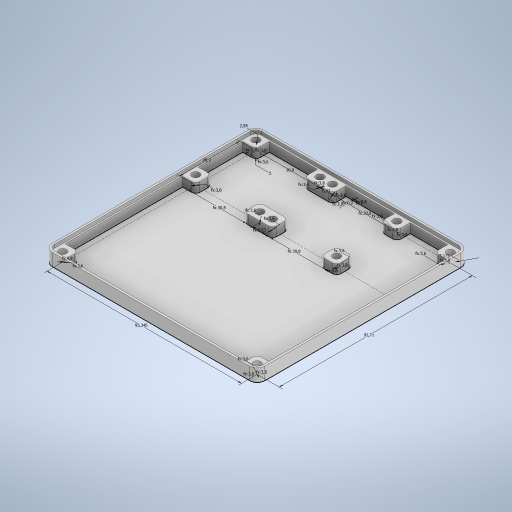
# Autodesk Inventor part: Housing_Bottom
Saved by Autodesk Inventor 2023 (Build 270158000, 158)
## iProperties
Created: 2023-02-18
Part Number: Housing_Bottom
Material: Generisch
Document SubType Name: Modeling
Designer: dvd62
Density: 1 g/cm^3
Appearance: Vorgabe
Author: dvd62
Autodesk Inventor part; units mm, degrees
ref_plane "YZ Plane" through (0, 0, 0) normal (1, 0, 0) x (0, 1, 0)
ref_plane "XZ Plane" through (0, 0, 0) normal (0, 1, 0) x (-1, 0, 0)
ref_plane "XY Plane" through (0, 0, 0) normal (0, 0, 1) x (1, 0, 0)
sketch "Skizze1" plane through (0, 0, 0) normal (0, 1, 0) x (-1, 0, 0)
  circle A0 centre (0, 0) radius 1.8
  line L0 (0, 0) -> (-93.345, 0) construction
  line L1 (-93.345, 0) -> (-93.345, -92.71) construction
  line L2 (-93.345, -92.71) -> (0, -92.71) construction
  line L3 (0, -92.71) -> (0, 0) construction
  circle A1 centre (0, -92.71) radius 1.8
  circle A2 centre (-93.345, -92.71) radius 1.8
  circle A3 centre (-93.345, 0) radius 1.8
  circle A4 centre (-30.8, -92.71) radius 1.8
  circle A5 centre (-36.83, -92.71) radius 1.8
  circle A6 centre (-67.63, -92.71) radius 1.8
  line L4 (0, -63.81) -> (-93.345, -63.81) construction
  circle A7 centre (0, -63.81) radius 1.8
  circle A8 centre (-30.8, -63.81) radius 1.8
  circle A9 centre (-36.83, -63.81) radius 1.8
  circle A10 centre (-67.63, -63.81) radius 1.8
  line L5 (0.635, -95.885) -> (-93.98, -95.885) construction
  line L6 (-96.52, -93.345) -> (-96.52, 0.635) construction
  line L7 (-93.98, 3.175) -> (0.635, 3.175) construction
  line L8 (3.175, 0.635) -> (3.175, -93.345) construction
  arc A11 (0.635, -95.885) -> (3.175, -93.345) centre (0.635, -93.345) ccw construction
  arc A12 (-96.52, -93.345) -> (-93.98, -95.885) centre (-93.98, -93.345) ccw construction
  arc A13 (-93.98, 3.175) -> (-96.52, 0.635) centre (-93.98, 0.635) ccw construction
  arc A14 (3.175, 0.635) -> (0.635, 3.175) centre (0.635, 0.635) ccw construction
  line L9 (-93.98, -96.085) -> (0.635, -96.085)
  arc A15 (0.635, -96.085) -> (3.375, -93.345) centre (0.635, -93.345) ccw
  line L10 (3.375, -93.345) -> (3.375, 0.635)
  arc A16 (3.375, 0.635) -> (0.635, 3.375) centre (0.635, 0.635) ccw
  line L11 (0.635, 3.375) -> (-93.98, 3.375)
  arc A17 (-93.98, 3.375) -> (-96.72, 0.635) centre (-93.98, 0.635) ccw
  line L12 (-96.72, 0.635) -> (-96.72, -93.345)
  arc A18 (-96.72, -93.345) -> (-93.98, -96.085) centre (-93.98, -93.345) ccw
  line L13 (0.635, -97.085) -> (-93.98, -97.085)
  arc A19 (-97.72, -93.345) -> (-93.98, -97.085) centre (-93.98, -93.345) ccw
  line L14 (-97.72, -93.345) -> (-97.72, 0.635)
  arc A20 (-93.98, 4.375) -> (-97.72, 0.635) centre (-93.98, 0.635) ccw
  line L15 (-93.98, 4.375) -> (0.635, 4.375)
  arc A21 (4.375, 0.635) -> (0.635, 4.375) centre (0.635, 0.635) ccw
  line L16 (4.375, 0.635) -> (4.375, -93.345)
  arc A22 (0.635, -97.085) -> (4.375, -93.345) centre (0.635, -93.345) ccw
  line L17 (0.635, -95.285) -> (-93.98, -95.285)
  arc A23 (-95.92, -93.345) -> (-93.98, -95.285) centre (-93.98, -93.345) ccw
  line L18 (-95.92, -93.345) -> (-95.92, 0.635)
  arc A24 (-93.98, 2.575) -> (-95.92, 0.635) centre (-93.98, 0.635) ccw
  line L19 (-93.98, 2.575) -> (0.635, 2.575)
  arc A25 (2.575, 0.635) -> (0.635, 2.575) centre (0.635, 0.635) ccw
  line L20 (2.575, 0.635) -> (2.575, -93.345)
  arc A26 (0.635, -95.285) -> (2.575, -93.345) centre (0.635, -93.345) ccw
  line L21 (-3.8, -95.285) -> (-3.8, -90.91)
  line L22 (-1.8, -88.91) -> (2.575, -88.91)
  line L23 (-27, -95.285) -> (-27, -90.91)
  line L24 (-29, -88.91) -> (-38.63, -88.91)
  line L25 (-40.63, -90.91) -> (-40.63, -95.285)
  line L26 (-63.83, -95.285) -> (-63.83, -90.91)
  line L27 (-65.83, -88.91) -> (-69.43, -88.91)
  line L28 (-71.43, -90.91) -> (-71.43, -95.285)
  line L29 (-89.545, -95.285) -> (-89.545, -90.91)
  line L30 (-91.545, -88.91) -> (-95.92, -88.91)
  line L31 (-95.92, -3.8) -> (-91.545, -3.8)
  line L32 (-89.545, -1.8) -> (-89.545, 2.575)
  line L33 (2.575, -3.8) -> (-1.8, -3.8)
  line L34 (-3.8, -1.8) -> (-3.8, 2.575)
  line L35 (2.575, -67.61) -> (-1.8, -67.61)
  line L36 (-3.8, -65.61) -> (-3.8, -62.01)
  line L37 (-1.8, -60.01) -> (2.575, -60.01)
  line L38 (-29, -67.61) -> (-38.63, -67.61)
  line L39 (-40.63, -65.61) -> (-40.63, -62.01)
  line L40 (-38.63, -60.01) -> (-29, -60.01)
  line L41 (-27, -62.01) -> (-27, -65.61)
  line L42 (-65.83, -67.61) -> (-69.43, -67.61)
  line L43 (-71.43, -65.61) -> (-71.43, -62.01)
  line L44 (-69.43, -60.01) -> (-65.83, -60.01)
  line L45 (-63.83, -62.01) -> (-63.83, -65.61)
  arc A27 (-1.8, -88.91) -> (-3.8, -90.91) centre (-1.8, -90.91) ccw
  arc A28 (-27, -90.91) -> (-29, -88.91) centre (-29, -90.91) ccw
  arc A29 (-38.63, -88.91) -> (-40.63, -90.91) centre (-38.63, -90.91) ccw
  arc A30 (-63.83, -90.91) -> (-65.83, -88.91) centre (-65.83, -90.91) ccw
  arc A31 (-69.43, -88.91) -> (-71.43, -90.91) centre (-69.43, -90.91) ccw
  arc A32 (-89.545, -90.91) -> (-91.545, -88.91) centre (-91.545, -90.91) ccw
  arc A33 (-65.83, -67.61) -> (-63.83, -65.61) centre (-65.83, -65.61) ccw
  arc A34 (-71.43, -65.61) -> (-69.43, -67.61) centre (-69.43, -65.61) ccw
  arc A35 (-69.43, -60.01) -> (-71.43, -62.01) centre (-69.43, -62.01) ccw
  arc A36 (-63.83, -62.01) -> (-65.83, -60.01) centre (-65.83, -62.01) ccw
  arc A37 (-27, -62.01) -> (-29, -60.01) centre (-29, -62.01) ccw
  arc A38 (-29, -67.61) -> (-27, -65.61) centre (-29, -65.61) ccw
  arc A39 (-40.63, -65.61) -> (-38.63, -67.61) centre (-38.63, -65.61) ccw
  arc A40 (-38.63, -60.01) -> (-40.63, -62.01) centre (-38.63, -62.01) ccw
  arc A41 (-1.8, -60.01) -> (-3.8, -62.01) centre (-1.8, -62.01) ccw
  arc A42 (-3.8, -65.61) -> (-1.8, -67.61) centre (-1.8, -65.61) ccw
  arc A43 (-3.8, -1.8) -> (-1.8, -3.8) centre (-1.8, -1.8) ccw
  arc A44 (-91.545, -3.8) -> (-89.545, -1.8) centre (-91.545, -1.8) ccw
  point P0 (-27, -67.61)
  point P1 (-40.63, -60.01)
  point P2 (-27, -60.01)
  dimension "d0" = 3.6
  dimension "d1" = 3.6
  dimension "d2" = 3.6
  dimension "d3" = 3.6
  dimension "d4" = 93.345
  dimension "d5" = 92.71
  dimension "d6" = 3.6
  dimension "d7" = 3.6
  dimension "d8" = 3.6
  dimension "d10" = 3.6
  dimension "d11" = 3.6
  dimension "d12" = 3.6
  dimension "d13" = 3.6
  dimension "d14" = 28.9
  dimension "d15" = 30.8
  dimension "d16" = 6.03
  dimension "d17" = 30.8
  dimension "d18" = 30.8
  dimension "d19" = 6.03
  dimension "d20" = 30.8
  dimension "d21" = 3.175
  dimension "d22" = 2.54
  dimension "d23" = 0.2
  dimension "d24" = 1
  dimension "d29" = 0.8
  dimension "d32" = 3.8
  dimension "d33" = 3.8
  dimension "d35" = 3.8
  dimension "d36" = 3.8
  dimension "d37" = 3.8
  dimension "d38" = 3.8
  dimension "d39" = 3.8
  dimension "d40" = 3.8
  dimension "d41" = 3.8
  dimension "d42" = 3.8
  dimension "d43" = 3.8
  dimension "d44" = 3.8
  dimension "d45" = 2
  constraints: 92 end point, 68 point on circle, 45 centre point, 44 tangent, 31 point on line, 21 perpendicular, 20 equal radius, 12 collinear, 12 parallel, 5 coincident, 4 horizontal, 3 vertical, 24 other
  measures "d0" diameter of A0
  measures "d1" diameter of A1
  measures "d2" diameter of A2
  measures "d3" diameter of A3
  measures "d4" distance of L0.start L0.end
  measures "d5" distance of L0.end L1.end
  measures "d6" diameter of A4
  measures "d7" diameter of A5
  measures "d8" diameter of A6
  measures "d10" diameter of A7
  measures "d11" diameter of A8
  measures "d12" diameter of A9
  measures "d13" diameter of A10
  measures "d14" distance between parallel lines of L2 L4
  measures "d15" distance of A4.centre A1.centre
  measures "d16" distance of A5.centre A4.centre
  measures "d17" distance of A6.centre A5.centre
  measures "d18" distance of A8.centre A7.centre
  measures "d19" distance of A8.centre A9.centre
  measures "d20" distance of A9.centre A10.centre
  measures "d21" distance between parallel lines of L5 L2
  measures "d22" radius of A11
  measures "d23" distance between parallel lines of L5 L9
  measures "d24" distance between parallel lines of L9 L13
  measures "d29" distance between parallel lines of L9 L17
  measures "d32" distance from line of A1.centre L21
  measures "d33" distance from line of A1.centre L22
  measures "d35" distance from line of L23 A4.centre
  measures "d36" distance from line of L25 A5.centre
  measures "d37" distance from line of L26 A6.centre
  measures "d38" distance from line of L28 A6.centre
  measures "d39" distance from line of L29 A2.centre
  measures "d40" distance from line of L42 A10.centre
  measures "d41" distance from line of L44 A10.centre
  measures "d42" distance from line of L33 L0.start
  measures "d43" distance from line of L32 A3.centre
  measures "d44" distance from line of L31 A3.centre
  measures "d45" radius of A27
extrude "Extrusion1" add sketch "Skizze1" against normal blind 1 contours A0 | A1 | A2 | A3 | A4 | A5 | A6 | A7 | A8 | A9 | A10 | A18 L12 A17 L11 A16 L10 A15 L9 | L13 A19 L14 A20 L15 A21 L16 A22 | L17 L21 A27 L22 L20 A26 | L17 L23 A28 L24 A29 L25 L26 A30 L27 A31 L28 L29 A32 L30 L18 L31 A44 L32 L19 L34 A43 L33 L20 L37 A41 L36 A42 L35 L22 A27 L21 | L17 L25 A29 L24 A28 L23 | L35 A42 L36 A41 L37 L20 | L17 L28 A31 L27 A30 L26 | L33 A43 L34 L19 A25 L20 | L17 A23 L18 L30 A32 L29 | L32 A44 L31 L18 A24 L19 | L38 A39 L39 A40 L40 A37 L41 A38 | L42 A34 L43 A35 L44 A36 L45 A33
extrude "Extrusion2" add sketch "Skizze1" along normal blind 6 contours L13 A19 L14 A20 L15 A21 L16 A22
extrude "Extrusion3" add sketch "Skizze1" along normal blind 4.4 contours A18 L12 A17 L11 A16 L10 A15 L9
extrude "Extrusion4" add sketch "Skizze1" along normal up to surface (4.4 mm away) contours L17 L21 A27 L22 L20 A26 | L17 L25 A29 L24 A28 L23 | L35 A42 L36 A41 L37 L20 | L17 L28 A31 L27 A30 L26 | L33 A43 L34 L19 A25 L20 | L17 A23 L18 L30 A32 L29 | L32 A44 L31 L18 A24 L19 | L38 A39 L39 A40 L40 A37 L41 A38 | L42 A34 L43 A35 L44 A36 L45 A33
chamfer "Fase1" distance 1 angle 45 8 edges at (97.72, -1, -46.355) (96.6246, -1, 3.2796) (46.6725, -1, 4.375) (-3.2796, -1, 3.2796) (-4.375, -1, -46.355) (-3.2796, -1, -95.9896) (46.6725, -1, -97.085) (96.6246, -1, -95.9896)
equation "\"d0\" = holeDim"
equation "\"d1\" = holeDim"
equation "\"d2\" = holeDim"
equation "\"d3\" = holeDim"
equation "\"d6\" = holeDim"
equation "\"d7\" = holeDim"
equation "\"d8\" = holeDim"
equation "\"d10\" = holeDim"
equation "\"d11\" = holeDim"
equation "\"d12\" = holeDim"
equation "\"d13\" = holeDim"
equation "\"d17\" = d15"
equation "\"d18\" = d15"
equation "\"d19\" = d16"
equation "\"d20\" = d15"
equation "\"d23\" = airGabWall"
equation "\"d24\" = topWallThick"
equation "\"d29\" = baseWallThick"
equation "\"d32\" = insertWallThick"
equation "\"d33\" = insertWallThick"
equation "\"d35\" = insertWallThick"
equation "\"d36\" = insertWallThick"
equation "\"d37\" = insertWallThick"
equation "\"d38\" = insertWallThick"
equation "\"d39\" = insertWallThick"
equation "\"d40\" = insertWallThick"
equation "\"d41\" = insertWallThick"
equation "\"d42\" = insertWallThick"
equation "\"d43\" = insertWallThick"
equation "\"d44\" = insertWallThick"
equation "\"d25\" = baseThick"
equation "\"d27\" = heightWall"
equation "\"d30\" = baseHeightWall"
equation "\"holeDim\" = 3.6"
equation "\"topWallThick\" = 1"
equation "\"airGabWall\" = 0.2"
equation "\"baseThick\" = 1"
equation "\"heightWall\" = heightInnerWall + pcbThick"
equation "\"baseWallThick\" = 0.8"
equation "\"pcbThick\" = 1.6"
equation "\"baseHeightWall\" = heightWall - pcbThick"
equation "\"heightInnerWall\" = 4.4"
equation "\"insertWallThick\" = 3.8"
